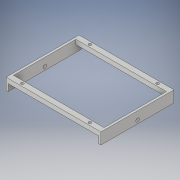
# Autodesk Inventor part: Fan-Holder-4355
Saved by Autodesk Inventor 2019 (Build 230136000, 136)
## iProperties
Created: 2019-02-01
Part Number: Fan-Holder-4355
Material: Generic
Document SubType Name: Modeling
Designer: bbramman
Density: 1 g/cm^3
Appearance: Default
Author: bbramman
Autodesk Inventor part; units mm, degrees
ref_plane "YZ Plane" through (0, 0, 0) normal (1, 0, 0) x (0, 1, 0)
ref_plane "XZ Plane" through (0, 0, 0) normal (0, 1, 0) x (-1, 0, 0)
ref_plane "XY Plane" through (0, 0, 0) normal (0, 0, 1) x (1, 0, 0)
sketch "Sketch1" plane through (0, 0, 0) normal (0, 1, 0) x (-1, 0, 0)
  line L0 (-53.34, 41) -> (53.34, 41)
  line L1 (53.34, 41) -> (53.34, -41)
  line L2 (53.34, -41) -> (-53.34, -41)
  line L3 (-53.34, -41) -> (-53.34, 41)
  line L4 (-53.34, 41) -> (53.34, -41) construction
  line L5 (53.34, 41) -> (-53.34, -41) construction
  line L6 (-50.8, 35) -> (50.8, 35)
  line L7 (50.8, 35) -> (50.8, -35)
  line L8 (50.8, -35) -> (-50.8, -35)
  line L9 (-50.8, -35) -> (-50.8, 35)
  line L10 (-50.8, 35) -> (50.8, -35) construction
  line L11 (50.8, 35) -> (-50.8, -35) construction
  point P0 (0, 0)
  dimension "d0" = 106.68
  dimension "d1" = 82
  dimension "d2" = 101.6
  dimension "d3" = 70
  constraints: 24 end point, 4 midpoint, 4 parallel, 2 horizontal, 2 perpendicular
  measures "d0" distance of L1.end L2.end
  measures "d1" distance of L0.end L1.end
  measures "d2" distance of L7.end L8.end
  measures "d3" distance of L6.end L7.end
extrude "Extrusion1" add sketch "Sketch1" along normal blind 5.08
sketch "Sketch2" plane through (0, 0, 0) normal (0, -1, 0) x (1, 0, 0)
  line L0 (-53.34, 41) -> (53.34, 41) projected
  line L1 (53.34, -41) -> (-53.34, -41) projected
  line L2 (53.34, 41) -> (50.7573, 41)
  line L3 (50.7573, 41) -> (50.7573, -41)
  line L4 (50.7573, -41) -> (53.34, -41)
  line L5 (53.34, -41) -> (53.34, 41)
  line L6 (-53.34, -41) -> (-50.8, -41)
  line L7 (-50.8, -41) -> (-50.8, 41)
  line L8 (-50.8, 41) -> (-53.34, 41)
  line L9 (-53.34, 41) -> (-53.34, -41)
  point P0 (0, 0)
  constraints: 16 end point, 4 parallel, 2 horizontal, 2 perpendicular, 2 point on line
extrude "Extrusion2" add sketch "Sketch2" along normal blind 7.62 contours L0 L7 L1 L9 | L0 L5 L1 L3
sketch "Sketch3" plane through (0, 5.08, 0) normal (0, 1, 0) x (1, 0, 0)
  line L0 (-40, -40) -> (40, -40)
  line L1 (40, -40) -> (40, 40)
  line L2 (40, 40) -> (-40, 40)
  line L3 (-40, 40) -> (-40, -40)
  line L4 (-40, -40) -> (40, 40) construction
  line L5 (40, -40) -> (-40, 40) construction
  line L6 (-40, 40) -> (-36.19, 40)
  line L7 (40, 40) -> (36.19, 40)
  line L8 (40, -40) -> (40, -36.19)
  line L9 (53.34, 41) -> (-53.34, 41) projected
  line L10 (-40, 41) -> (-40, 35)
  line L11 (50.7573, 35) -> (-50.8, 35) projected
  point P0 (0, 0)
  point P1 (-38, 38)
  point P2 (-38, -38)
  point P3 (38, -38)
  point P4 (38, 38)
  dimension "d8" = 80
  dimension "d9" = 80
  dimension "d10" = 3.81
  constraints: 20 end point, 10 point on line, 2 midpoint, 2 parallel, 1 horizontal, 1 perpendicular
  measures "d8" distance of L2.end L1.end
  measures "d9" distance of L1.end L0.end
  measures "d10" distance of L2.end L6.end
hole "Hole1" at (-38, 5.08, -38) at (38, 5.08, -38) at (38, 5.08, 38) at (-38, 5.08, 38) direction (0, -1, 0) diameter 3.048 end through all
sketch "Sketch4" plane through (53.34, 5.08, 41) normal (1, 0, 0) x (0, 0, -1)
  line L0 (6, -5.08) -> (0, -5.08) projected
  line L1 (0, -12.7) -> (0, 0) projected
  line L2 (0, -5.08) -> (0, -12.7)
  line L3 (0, -12.7) -> (0, -8.89)
  line L4 (0, -8.89) -> (82, -8.89)
  point P0 (41, -5.08)
  point P1 (82, -5.08)
  point P2 (82, -12.7)
  point P3 (41, -8.89)
  constraints: 6 end point, 2 midpoint, 1 collinear, 1 horizontal
hole "Hole2" at (53.34, -3.81, 0) direction (-1, 0, 0) diameter 3.81 end through all
body "Solid1"
